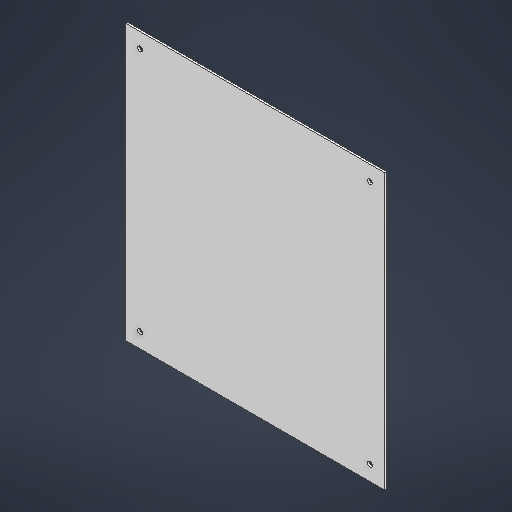
# Autodesk Inventor part: PlaqueArmoire
Saved by Autodesk Inventor 2026.2 (Build 302298010, 298A)
## iProperties
Created: 2026-05-13
Part Number: PlaqueArmoire
Material: Générique
Document SubType Name: Modeling
Designer: romai
Density: 1 g/cm^3
Appearance: Par défaut
Author: romai
Autodesk Inventor part; units mm, degrees
ref_plane "YZ Plane" through (0, 0, 0) normal (1, 0, 0) x (0, 1, 0)
ref_plane "XZ Plane" through (0, 0, 0) normal (0, 1, 0) x (-1, 0, 0)
ref_plane "XY Plane" through (0, 0, 0) normal (0, 0, 1) x (1, 0, 0)
sketch "Esquisse1" plane through (0, 0, 0) normal (0, 0, 1) x (1, 0, 0)
  line L0 (-130, 137.5) -> (130, 137.5)
  line L1 (130, 137.5) -> (130, -137.5)
  line L2 (130, -137.5) -> (-130, -137.5)
  line L3 (-130, -137.5) -> (-130, 137.5)
  line L4 (-130, 137.5) -> (130, -137.5) construction
  line L5 (130, 137.5) -> (-130, -137.5) construction
  line L6 (-117.5, -125) -> (117.5, -125)
  line L7 (117.5, -125) -> (117.5, 125)
  line L8 (117.5, 125) -> (-117.5, 125)
  line L9 (-117.5, 125) -> (-117.5, -125)
  line L10 (-117.5, -125) -> (117.5, 125) construction
  line L11 (117.5, -125) -> (-117.5, 125) construction
  circle A0 centre (-115, 122.5) radius 2.5
  circle A1 centre (115, 122.5) radius 2.5
  circle A2 centre (-115, -122.5) radius 2.5
  circle A3 centre (115, -122.5) radius 2.5
  point P0 (0, 0)
  dimension "d0" = 260
  dimension "d1" = 275
  dimension "d2" = 12.5
  dimension "d3" = 12.5
  dimension "d4" = 5
  dimension "d5" = 5
  dimension "d6" = 5
  dimension "d7" = 5
  constraints: 24 end point, 8 tangent, 4 centre point, 4 midpoint, 4 parallel, 2 horizontal, 2 perpendicular
  measures "d0" distance of L1.end L2.end
  measures "d1" distance of L0.end L1.end
  measures "d2" distance between parallel lines of L1 L7
  measures "d3" distance between parallel lines of L0 L8
  measures "d4" diameter of A0
  measures "d5" diameter of A1
  measures "d6" diameter of A2
  measures "d7" diameter of A3
extrude "Extrusion1" add sketch "Esquisse1" along normal blind 2 contours L0 L1 L2 L3 | L9 A2 L6 | A2 L9 A0 L8 A1 L7 A3 L6 | A3 L7 L6 | L9 L8 A0 | A1 L8 L7
